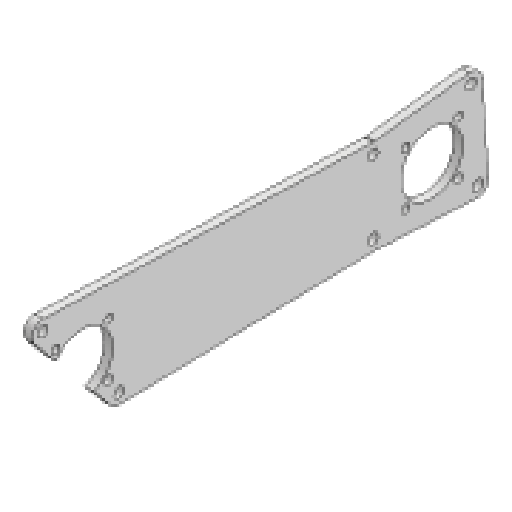
# Autodesk Inventor part: ChassiMotorMount3.3
Saved by Autodesk Inventor 2023 (Build 270158000, 158)
## iProperties
Created: 2022-09-16
Part Number: ChassiMotorMount3.3
Material: Generic
Document SubType Name: Modeling
Designer: deli
Density: 1 g/cm^3
Appearance: Default
Author: deli
Autodesk Inventor part; units mm, degrees
ref_plane "YZ Plane" through (0, 0, 0) normal (1, 0, 0) x (0, 1, 0)
ref_plane "XZ Plane" through (0, 0, 0) normal (0, 1, 0) x (-1, 0, 0)
ref_plane "XY Plane" through (0, 0, 0) normal (0, 0, 1) x (1, 0, 0)
sketch "Sketch1" plane through (0, 0, 0) normal (1, 0, 0) x (0, 1, 0)
  circle A0 centre (39.7366, 73.6498) radius 2
  circle A1 centre (5.9097, 76.131) radius 2
  circle A2 centre (8.0238, -49.5013) radius 2
  circle A3 centre (5.9097, -88.4471) radius 2
  circle A4 centre (39.7366, -85.9659) radius 2
  arc A5 (43.7073, 73.1662) -> (40.0292, 77.6391) centre (39.7366, 73.6498) ccw
  circle A6 centre (35.2955, -49.5013) radius 4 construction
  arc A7 (40.0292, -89.9552) -> (43.7073, -85.4823) centre (39.7366, -85.9659) ccw
  arc A8 (1.9155, -88.2303) -> (6.2023, -92.4364) centre (5.9097, -88.4471) ccw
  arc A9 (6.2023, 80.1203) -> (1.9155, 75.9142) centre (5.9097, 76.131) ccw
  line L0 (4.0297, -49.2844) -> (1.9155, -88.2303)
  line L1 (40.0292, 77.6391) -> (6.2023, 80.1203)
  line L2 (40.0292, -89.9552) -> (6.2023, -92.4364)
  line L3 (43.7073, -85.4823) -> (39.2662, -49.0177)
  circle A10 centre (21.6597, -71.3445) radius 11.5
  circle A11 centre (11.7602, -61.445) radius 1.6
  circle A12 centre (31.5592, -61.445) radius 1.6
  circle A13 centre (31.5592, -81.244) radius 1.6
  circle A14 centre (11.7602, -81.244) radius 1.6
  line L4 (31.5592, -61.445) -> (31.5592, -81.244) construction
  line L5 (31.5592, -81.244) -> (11.7602, -81.244) construction
  line L6 (11.7602, -81.244) -> (11.7602, -61.445) construction
  line L7 (11.7602, -61.445) -> (31.5592, -61.445) construction
  line L8 (11.7602, -81.244) -> (31.5592, -61.445) construction
  line L9 (11.7602, -61.445) -> (31.5592, -81.244) construction
  circle A15 centre (35.2955, -49.5013) radius 2
  circle A16 centre (39.7366, 73.6498) radius 2 projected
  circle A17 centre (21.6597, 59.0284) radius 4 projected
  circle A18 centre (21.6597, -71.3445) radius 4 projected
  circle A19 centre (5.9097, -88.4471) radius 2 projected
  circle A20 centre (39.7366, -85.9659) radius 2 projected
  circle A21 centre (35.2955, -49.5013) radius 2 projected
  circle A22 centre (8.0238, -49.5013) radius 2 projected
  circle A23 centre (5.9097, 76.131) radius 2 projected
  circle A24 centre (35.2955, 37.1852) radius 2 projected
  circle A25 centre (35.8305, -6.158) radius 2 projected
  circle A26 centre (8.0238, 37.1852) radius 2 projected
  circle A27 centre (21.6597, 15.342) radius 4 projected
  circle A28 centre (7.4888, -6.158) radius 2 projected
  circle A29 centre (21.6597, -27.658) radius 4 projected
  circle A30 centre (35.2955, 37.1852) radius 4 construction
  arc A31 (39.8302, -6.2074) -> (39.8302, -6.1087) centre (35.8305, -6.158) ccw
  arc A32 (3.4891, -6.1087) -> (3.4891, -6.2074) centre (7.4888, -6.158) ccw
  circle A33 centre (8.0238, 37.1852) radius 4 construction
  circle A34 centre (21.6597, 59.0284) radius 11.5
  circle A35 centre (31.5592, 68.9279) radius 1.6
  circle A36 centre (31.5592, 49.1289) radius 1.6
  circle A37 centre (11.7602, 49.1289) radius 1.6
  circle A38 centre (11.7602, 68.9279) radius 1.6
  line L10 (31.5592, 68.9279) -> (31.5592, 49.1289) construction
  line L11 (31.5592, 49.1289) -> (11.7602, 49.1289) construction
  line L12 (11.7602, 49.1289) -> (11.7602, 68.9279) construction
  line L13 (11.7602, 68.9279) -> (31.5592, 68.9279) construction
  line L14 (31.5592, 68.9279) -> (11.7602, 49.1289) construction
  line L15 (11.7602, 68.9279) -> (31.5592, 49.1289) construction
  circle A39 centre (29.6597, 23.342) radius 2
  circle A40 centre (29.6597, 7.342) radius 2
  circle A41 centre (13.6597, 7.342) radius 2
  circle A42 centre (13.6597, 23.342) radius 2
  line L16 (29.6597, 23.342) -> (29.6597, 7.342) construction
  line L17 (29.6597, 7.342) -> (13.6597, 7.342) construction
  line L18 (13.6597, 7.342) -> (13.6597, 23.342) construction
  line L19 (13.6597, 23.342) -> (29.6597, 23.342) construction
  line L20 (29.6597, 23.342) -> (13.6597, 7.342) construction
  line L21 (13.6597, 23.342) -> (29.6597, 7.342) construction
  circle A43 centre (13.6597, -35.658) radius 2
  line L22 (13.6597, -35.658) -> (13.6597, -19.658) construction
  circle A44 centre (13.6597, -19.658) radius 2
  line L23 (29.6597, -35.658) -> (13.6597, -35.658) construction
  circle A45 centre (29.6597, -35.658) radius 2
  line L24 (29.6597, -19.658) -> (29.6597, -35.658) construction
  line L25 (29.6597, -19.658) -> (13.6597, -35.658) construction
  line L26 (13.6597, -19.658) -> (29.6597, -35.658) construction
  line L27 (13.6597, -19.658) -> (29.6597, -19.658) construction
  circle A46 centre (29.6597, -19.658) radius 2
  line L28 (43.7073, 73.1662) -> (39.2662, 36.7016)
  line L29 (39.2952, 37.2345) -> (39.8302, -6.1087)
  line L30 (39.8302, -6.2074) -> (39.2952, -49.5506)
  line L31 (3.4891, -6.1087) -> (4.0241, 37.2345)
  line L32 (4.0297, 36.9683) -> (1.9155, 75.9142)
  line L33 (3.4891, -6.2074) -> (4.0241, -49.5506)
  circle A47 centre (8.0238, -49.5013) radius 4 construction
  point P0 (0, 0)
  point P1 (21.0827, -58.3908)
  point P2 (53.615, -21.1734)
  point P3 (53.7299, -25.9433)
  point P4 (-6.0389, 43.0405)
  point P5 (-46.726, 40.7276)
  point P6 (4.0225, 37.1013)
  point P7 (4.0225, -49.4174)
  point P8 (39.2985, -49.2832)
  point P9 (39.2985, 36.9671)
  point P10 (14.7045, 49.87)
  point P11 (12.5013, 52.0732)
  dimension "d0" = 8
  dimension "d1" = 8
  dimension "d3" = 8
  dimension "d4" = 8
  dimension "d5" = 8
  dimension "d16" = 3.2
  dimension "d17" = 3.2
  dimension "d18" = 3.2
  dimension "d19" = 3.2
  dimension "d23" = 28
  dimension "d24" = 4
  dimension "d25" = 23
  dimension "d26" = 3.2
  dimension "d27" = 3.2
  dimension "d28" = 3.2
  dimension "d29" = 3.2
  dimension "d30" = 28
  dimension "d38" = 4
  dimension "d44" = 16
  constraints: 68 end point, 34 centre point, 20 point on circle, 20 tangent, 18 equal radius, 12 coincident, 9 concentric, 9 perpendicular, 8 vertical, 6 midpoint, 4 equal length, 2 point on line
  measures "d0" diameter of A5
  measures "d1" diameter of A9
  measures "d3" diameter of A6
  measures "d4" diameter of A7
  measures "d5" diameter of A8
  measures "d16" diameter of A11
  measures "d17" diameter of A12
  measures "d18" diameter of A13
  measures "d19" diameter of A14
  measures "d23" distance of L5.end L4.start
  measures "d24" diameter of A0
  measures "d25" diameter of A34
  measures "d26" diameter of A35
  measures "d27" diameter of A36
  measures "d28" diameter of A37
  measures "d29" diameter of A38
  measures "d30" distance of L10.start L12.start
  measures "d38" diameter of A46
  measures "d44" distance of L24.start L23.start
extrude "Extrusion1" add sketch "Sketch1" along normal blind 3.175 contours L28 L29 A31 L30 L3 A7 L2 A8 L0 L33 A32 L31 L32 A9 L1 A5
fillet "Fillet1" radius 4.7625 4 edges at (1.5875, 39.2985, 36.9671) (1.5875, 39.2985, -49.2832) (1.5875, 4.0225, 37.1013) (1.5875, 4.0225, -49.4174)
equation "\"d1\" = d0"
equation "\"d3\" = d0"
equation "\"d4\" = d0"
equation "\"d5\" = d0"
equation "\"d16\" = d12"
equation "\"d17\" = d12"
equation "\"d18\" = d12"
equation "\"d19\" = d12"
equation "\"d23\" = d20"
equation "\"d12\" = 3.2"
equation "\"d20\" = 28"
body "Solid1"
